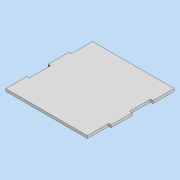
# Autodesk Inventor part: simple wall test
Saved by Autodesk Inventor 2020 (Build 240168000, 168)
## iProperties
Created: 2020-12-17
Part Number: simple wall test
Material: Generic
Document SubType Name: Modeling
Designer: solar
Density: 1 g/cm^3
Appearance: Default
Author: solar
Autodesk Inventor part; units mm, degrees
ref_plane "YZ Plane" through (0, 0, 0) normal (1, 0, 0) x (0, 1, 0)
ref_plane "XZ Plane" through (0, 0, 0) normal (0, 1, 0) x (-1, 0, 0)
ref_plane "XY Plane" through (0, 0, 0) normal (0, 0, 1) x (1, 0, 0)
sketch "Sketch1" plane through (0, 0, 0) normal (0, 1, 0) x (-1, 0, 0)
  line L0 (100, 100.3504) -> (-94, 100.3504)
  line L1 (94, -100) -> (94, -50)
  line L2 (94, -50) -> (100, -50)
  line L3 (100, 0) -> (94, 0)
  line L4 (-100, -50) -> (-94, -50)
  line L5 (-94, -50) -> (-94, 0)
  line L6 (-94, 0) -> (-100, 0)
  line L7 (94, 0) -> (94, 50)
  line L8 (94, 50) -> (100, 50)
  line L9 (94, 0) -> (100, 0)
  line L10 (-100, 50) -> (-94, 50)
  line L11 (-94, 50) -> (-94, 100.3504)
  line L12 (94, -100) -> (-100, -100)
  line L13 (100, -50) -> (100, 0)
  line L14 (100, 50) -> (100, 100.3504)
  line L15 (-100, 50) -> (-100, 0)
  line L16 (-100, -50) -> (-100, -100)
  point P0 (0, 0)
  dimension "d23" = 50
  dimension "d25" = 6
  dimension "d26" = 50
  dimension "d27" = 50
  constraints: 35 end point, 11 perpendicular, 8 parallel, 3 horizontal, 1 collinear
  measures "d23" distance of L1.start L1.end
  measures "d25" distance of L4.start L4.end
  measures "d26" distance of L4.end L5.end
  measures "d27" distance of L3.end L7.end
extrude "Extrusion2" add sketch "Sketch1" along normal blind 6
body "Solid2"
